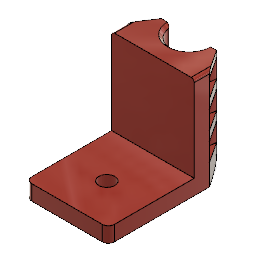
Cable_mount v9 (Autodesk Fusion 360 design; units mm, degrees)
Autodesk Fusion 360 part; units mm, degrees
sketch "Sketch1" plane through (0, 0, 0) normal (0, 1, 0) x (1, 0, 0)
  line L0 (-13.5, 0) -> (13.5, 0)
  line L1 (13.5, 0) -> (13.5, -28)
  line L2 (13.5, -28) -> (-13.5, -28)
  line L3 (-13.5, -28) -> (-13.5, 0)
  line L4 (-13.5, 0) -> (13.5, 0)
  line L5 (13.5, 0) -> (13.5, 5)
  line L6 (13.5, 5) -> (-13.5, 5)
  line L7 (-13.5, 5) -> (-13.5, 0)
  line L8 (0, 0) -> (0, 28) construction
  circle A0 centre (0, 11.8) radius 6
  circle A1 centre (0, 11.8) radius 9
  line L9 (9, 11.8) -> (-9, 11.8)
  line L10 (-9, 11.8) -> (-13.5, 5)
  line L11 (9, 11.8) -> (13.5, 5)
  circle A2 centre (0, 11.8) radius 11
  line L12 (-13.5, 5) -> (-3.7551, 1.4608)
  line L13 (13.5, 5) -> (3.7551, 1.4608)
  point P0 (0, 2.8)
  point P1 (0, 0.8)
  dimension "d1" = 5
  dimension "d2" = 28
  dimension "d10" = 12
  dimension "d11" = 18
  dimension "d47" = 22
  dimension "d48" = 0.8
  dimension "d49" = 27
  constraint horizontal L0
  constraint vertical L1
  constraint horizontal L2
  constraint vertical L3
  constraint coincident L8.start L0
  constraint horizontal L4
  constraint vertical L5
  constraint horizontal L6
  constraint vertical L7
  constraint coincident L8.start origin
  constraint perpendicular L4 L8
  constraint coincident L8 A0.centre
  constraint concentric A0 A1
  constraint collinear L1 L5
  constraint coincident A1 L9.start
  constraint coincident A1 L9.end
  constraint perpendicular L8 L9
  constraint coincident A0.centre L9
  constraint coincident L8 P0
  constraint coincident A1 P0
  constraint coincident L6 L7.start
  constraint coincident L6 L5.end
  constraint concentric A0 A2
  constraint coincident L8 P1
  constraint coincident A2 P1
  constraint coincident L6.end L7.start
  constraint coincident L5.end L6.start
  constraint coincident A2 L12.end
  constraint tangent A2 L12
  constraint coincident A2 L13.end
  constraint tangent A2 L13
  constraint midpoint L8.start L4
  measures "d1" distance of L0.end L5.end
  measures "d2" distance of L0.end L1.end
  measures "d10" diameter of A0
  measures "d11" diameter of A1
  measures "d47" diameter of A2
  measures "d48" distance of L4 P1
  measures "d49" distance of L1.end L2.end
extrude "Extrude1" add sketch "Sketch1" along normal blind 5 contours L0 L1 L2 L3 L4
extrude "Extrude2" add sketch "Sketch1" along normal blind 5 and the other way blind 28 contours L0 L4 L5 L7 A2 L12 L13 | L6 L10 A2 | L6 A2 L12 | L6 A2 L13 | L6 L11 A2 | L6 A1 L10 A2 | L6 A1 A2 | L6 A1 L11 A2 | L6 A0 A1 L9 | L6 A1
extrude "Extrude3" cut sketch "Sketch1" against normal blind 6 from surface at -2 contours L6 L10 A2 | L6 A2 L12 | L6 A2 L13 | L6 L11 A2 | L6 A1 L10 A2 | L6 A1 A2 | L6 A1 L11 A2
extrude "Extrude4" cut sketch "Sketch1" along normal blind 6 from surface at -26 contours L6 L10 A2 | L6 A2 L12 | L6 A2 L13 | L6 L11 A2 | L6 A1 L10 A2 | L6 A1 A2 | L6 A1 L11 A2
extrude "Extrude8" cut sketch "Sketch1" against normal blind 6 from surface at -11 contours L6 L10 A2 | L6 A2 L12 | L6 A2 L13 | L6 L11 A2 | L6 A1 L10 A2 | L6 A1 A2 | L6 A1 L11 A2
fillet "Fillet1" radius 8 1 edges at (0, 5, -5.8)
sketch "Sketch3" plane through (0, 0, 0) normal (0, 1, 0) x (1, 0, 0)
  line L0 (0, -28) -> (0, 0) construction
  circle A0 centre (0, -15) radius 2.6
  dimension "d32" = 5.2
  dimension "d46" = 15
  constraint coincident L0.end origin
  constraint vertical L0
  constraint coincident L0 A0.centre
  measures "d32" diameter of A0
  measures "d46" distance of A0.centre L0.end
extrude "Extrude7" cut sketch "Sketch3" along normal through all
fillet "Fillet2" radius 2 2 edges at (13.5, 2.5, 28) (-13.5, 2.5, 28)
fillet "Fillet2" radius 1 2 edges at (-13.5, -28, -2.5) (13.5, -28, -2.5)
fillet "Fillet3" radius 1 4 edges at (6, -15.5, -11.8) (6.7889, 0.4641, -11.8) (-6, -15.5, -11.8) (-6.7889, 0.4641, -11.8)
chamfer "Chamfer1" distance 1 angle 45 1 edges at (0, -28, -5.8) tangent chain off
move_body "Move1" bodies 1 to x (-1, 0, 0) y (0, -1, 0) z (0, 0, 1) at (0, 0, 0)
equation "d11 = d10 + ( 2 * 3 ) * 1 mm"
equation "d47 = d11 + ( 2 * 2 ) * 1 mm"
